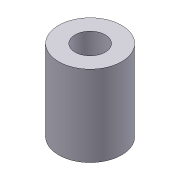
# Autodesk Inventor part: standoff815mm
Saved by Autodesk Inventor 2014 SP1 (Build 180222100, 222)
## iProperties
Created: 2011-03-09
Part Number: standoff815mm
Material: Aluminum-6061
Document SubType Name: Modeling
Designer: Robert Davis
Mass: 0.438627 g
Surface Area: 2.71685 cm^2
Volume: 0.161855 cm^3
Density: 2.71 g/cm^3
Description: AL SPACER
Appearance: Aluminum - Flat
Author: Robert Davis
Autodesk Inventor part; units mm, degrees
ref_plane "YZ Plane" through (0, 0, 0) normal (1, 0, 0) x (0, 1, 0)
ref_plane "XZ Plane" through (0, 0, 0) normal (0, 1, 0) x (-1, 0, 0)
ref_plane "XY Plane" through (0, 0, 0) normal (0, 0, 1) x (1, 0, 0)
sketch "Sketch1" plane through (0, 0, 0) normal (0, 0, 1) x (1, 0, 0)
  circle A0 centre (0, 0) radius 1.524
  circle A1 centre (0, 0) radius 3.175
  dimension "d0" = 6.35
  dimension "d1" = 3.048
  constraints: 2 centre point
  measures "d0" diameter of A1
  measures "d1" diameter of A0
extrude "Extrusion1" add sketch "Sketch1" along normal mid plane 8.15
body "Solid1"
